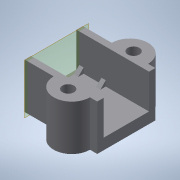
# Autodesk Inventor part: Лайн-райсер крепление моторов-основа версия 3
Saved by Autodesk Inventor 2020 (Build 240168000, 168)
## iProperties
Created: 2016-03-20
Part Number: Лайн-райсер крепление моторов-основа версия 3
Material: Типовые
Document SubType Name: Modeling
Designer: Романько Павел
Density: 1 g/cm^3
Appearance: По умолчанию
Author: Романько Павел
Autodesk Inventor part; units mm, degrees
ref_plane "YZ Plane" through (0, 0, 0) normal (1, 0, 0) x (0, 1, 0)
ref_plane "XZ Plane" through (0, 0, 0) normal (0, 1, 0) x (-1, 0, 0)
ref_plane "XY Plane" through (0, 0, 0) normal (0, 0, 1) x (1, 0, 0)
sketch "Эскиз1" plane through (0, 0, 0) normal (0, 0, 1) x (1, 0, 0)
  line L0 (10, 8) -> (10, -8)
  line L1 (-10, -8) -> (-10, 8)
  line L2 (-10, 8) -> (10, -8) construction
  line L3 (10, 8) -> (-10, -8) construction
  line L4 (3, 13.7772) -> (3, -20.7118) construction
  circle A0 centre (3, 0) radius 9 construction
  circle A1 centre (3, 9) radius 1.6
  circle A2 centre (3, -9) radius 1.6
  arc A3 (8, 8) -> (-2, 8) centre (3, 8) ccw
  arc A4 (-2, -8) -> (8, -8) centre (3, -8) ccw
  line L5 (-10, 8) -> (-2, 8)
  line L6 (8, 8) -> (10, 8)
  line L7 (10, -8) -> (8, -8)
  line L8 (-2, -8) -> (-10, -8)
  point P0 (0, 0)
  dimension "d0" = 20
  dimension "d1" = 16
  dimension "d2" = 13
  dimension "d3" = 18
  dimension "d4" = 3.2
  dimension "d5" = 3.2
  dimension "d6" = 5
  dimension "d7" = 5
  dimension "d19" = 7
  constraints: 18 end point, 6 point on circle, 5 centre point, 5 parallel, 5 point on line, 2 horizontal, 2 midpoint, 2 perpendicular, 1 vertical
  measures "d0" distance of L0.end L1.start
  measures "d1" distance of L0.start L0.end
  measures "d2" distance between parallel lines of L1 L4
  measures "d3" diameter of A0
  measures "d4" diameter of A1
  measures "d5" diameter of A2
  measures "d6" radius of A3
  measures "d7" radius of A4
  measures "d19" distance from line of L0 A1.centre
extrude "Выдавливание1" add sketch "Эскиз1" along normal blind 12.5
sketch "Эскиз2" plane through (0, 0, 12.5) normal (0, 0, 1) x (1, 0, 0)
  line L0 (10, -8) -> (10, 8) projected
  line L1 (-10, 6.25) -> (10, 6.25)
  line L2 (10, 6.25) -> (10, -6.25)
  line L3 (10, -6.25) -> (-10, -6.25)
  line L4 (-10, -6.25) -> (-10, 6.25)
  line L5 (-10, 6.25) -> (10, -6.25) construction
  line L6 (10, 6.25) -> (-10, -6.25) construction
  point P0 (0, 0)
  dimension "d10" = 12.5
  constraints: 12 end point, 2 equal length, 2 midpoint, 1 horizontal, 1 parallel, 1 point on line
  measures "d10" distance of L1.end L2.end
extrude "Выдавливание2" cut sketch "Эскиз2" against normal blind 9.5
sketch "Эскиз3" plane through (0, 0, 0) normal (0, 0, -1) x (-1, 0, 0)
  circle A0 centre (-3, -9) radius 1.6 projected
  circle A1 centre (-3, 9) radius 1.6 projected
  line L0 (10, 8) -> (10, -8) projected
  line L1 (2, 8) -> (10, 8) projected
  arc A2 (2, 8) -> (-8, 8) centre (-3, 8) ccw projected
  line L2 (-10, 8) -> (-8, 8) projected
  line L3 (-10, -8) -> (-10, 8) projected
  line L4 (-8, -8) -> (-10, -8) projected
  arc A3 (-8, -8) -> (2, -8) centre (-3, -8) ccw projected
  line L5 (10, -8) -> (2, -8) projected
  line L6 (-3, -12.4064) -> (-5.95, -10.7032)
  line L7 (-5.95, -10.7032) -> (-5.95, -7.2968)
  line L8 (-5.95, -7.2968) -> (-3, -5.5936)
  line L9 (-3, -5.5936) -> (-0.05, -7.2968)
  line L10 (-0.05, -7.2968) -> (-0.05, -10.7032)
  line L11 (-0.05, -10.7032) -> (-3, -12.4064)
  circle A4 centre (-3, 9) radius 1.6 projected
  line L12 (-3, 5.5936) -> (-5.95, 7.2968)
  line L13 (-5.95, 7.2968) -> (-5.95, 10.7032)
  line L14 (-5.95, 10.7032) -> (-3, 12.4064)
  line L15 (-3, 12.4064) -> (-0.05, 10.7032)
  line L16 (-0.05, 10.7032) -> (-0.05, 7.2968)
  line L17 (-0.05, 7.2968) -> (-3, 5.5936)
  point P0 (0, 0)
  dimension "d20" = 5.9
  dimension "d21" = 5.9
  constraints: 24 end point, 2 coincident, 26 other
  measures "d20" distance between parallel lines of L14 L17
  measures "d21" distance between parallel lines of L9 L6
extrude "Выдавливание3" cut sketch "Эскиз3" against normal blind 1.5 contours L6 L7 L8 L9 L10 L11 | L12 L13 L14 L15 L16 L17
ref_plane "РабПлоскость1" through (-9.2, -8, 0) normal (-1, 0, 0) x (0, 0, 1)
sketch "Эскиз4" plane through (-9.2, -8, 0) normal (-1, 0, 0) x (0, 0, 1)
  line L0 (4.5, 18.54) -> (4.5, -1.8097) construction
  line L1 (6.9459, 12.75) -> (1.1069, 12.75) construction
  line L2 (6.9459, 3.25) -> (1.1069, 3.25) construction
  line L3 (3, 14.25) -> (3, 1.75) construction
  line L4 (12.5, 14.25) -> (3, 14.25) construction
  line L5 (3, 1.75) -> (12.5, 1.75) construction
  line L6 (3, 14.25) -> (4.5, 14.25)
  line L7 (3, 14.25) -> (3, 12.75)
  line L8 (3, 12.75) -> (4.5, 14.25)
  line L9 (3, 3.25) -> (3, 1.75)
  line L10 (3, 1.75) -> (4.5, 1.75)
  line L11 (3, 3.25) -> (4.5, 1.75)
  point P0 (0, 8)
  dimension "d25" = 1.5
  dimension "d26" = 1.5
  dimension "d27" = 1.5
  constraints: 18 end point, 8 point on line, 2 horizontal, 1 collinear, 1 vertical
  measures "d25" distance between parallel lines of L3 L0
  measures "d26" distance between parallel lines of L4 L1
  measures "d27" distance between parallel lines of L2 L5
extrude "Выдавливание4" add sketch "Эскиз4" against normal blind 1.2
pattern_linear "Прямоуг.массив1" count 2 spacing 6.1 along (1, 0, 0) of "Выдавливание4"
